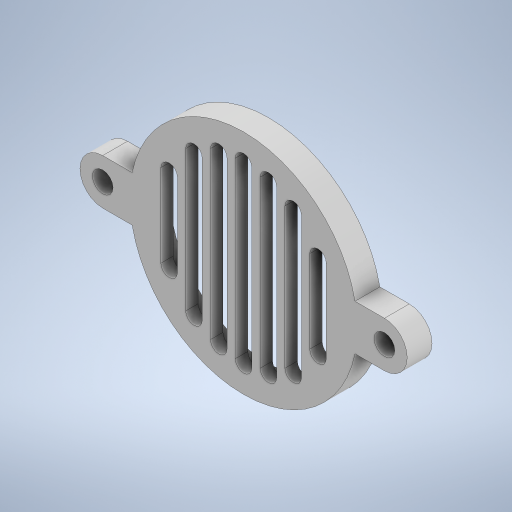
# Autodesk Inventor part: 스피커 홀더
Saved by Autodesk Inventor 2023 (Build 270158000, 158)
## iProperties
Created: 2022-11-10
Part Number: 스피커 홀더
Material: 일반
Document SubType Name: Modeling
Designer: user
Density: 1 g/cm^3
Appearance: 기본값
Author: user
Autodesk Inventor part; units mm, degrees
ref_plane "YZ Plane" through (0, 0, 0) normal (1, 0, 0) x (0, 1, 0)
ref_plane "XZ Plane" through (0, 0, 0) normal (0, 1, 0) x (-1, 0, 0)
ref_plane "XY Plane" through (0, 0, 0) normal (0, 0, 1) x (1, 0, 0)
sketch "스케치1" plane through (0, 0, 0) normal (0, 0, 1) x (1, 0, 0)
  circle A0 centre (0, 0) radius 13.75
  circle A1 centre (17.0329, 0) radius 1.25
  circle A2 centre (17.0329, 0) radius 2.75
  line L0 (17.0329, 2.75) -> (13.4722, 2.75)
  line L1 (17.0329, -2.75) -> (13.4722, -2.75)
  line L2 (0, 0) -> (0, 3.2191)
  circle A3 centre (-17.0329, 0) radius 1.25
  circle A4 centre (-17.0329, 0) radius 2.75
  line L3 (-17.0329, 2.75) -> (-13.4722, 2.75)
  line L4 (-17.0329, -2.75) -> (-13.4722, -2.75)
  dimension "d0" = 27.5
  dimension "d1" = 2.5
  dimension "d2" = 5.5
  constraints: 10 end point, 6 point on circle, 6 symmetric about line, 5 centre point, 3 coincident, 1 horizontal, 1 vertical, 2 other
  measures "d0" diameter of A0
  measures "d1" diameter of A1
  measures "d2" diameter of A2
extrude "돌출1" add sketch "스케치1" along normal blind 3
sketch "스케치2" plane through (0, 0, 0) normal (0, 0, -1) x (-1, 0, 0)
  circle A0 centre (0, 0) radius 12
  dimension "d5" = 24
  constraints: 1 centre point, 1 coincident
  measures "d5" diameter of A0
extrude "돌출2" cut sketch "스케치2" against normal blind 1.5
sketch "스케치3" plane through (0, 0, 1.5) normal (0, 0, -1) x (-1, 0, 0)
  line L0 (0, 10.5) -> (0, -10.5) construction
  line L1 (-1, 10.5) -> (-1, -10.5)
  line L2 (1, -10.5) -> (1, 10.5)
  arc A0 (1, 10.5) -> (-1, 10.5) centre (0, 10.5) ccw
  arc A1 (-1, -10.5) -> (1, -10.5) centre (0, -10.5) ccw
  line L3 (3, -10) -> (3, 10) construction
  line L4 (4, -10) -> (4, 10)
  line L5 (2, 10) -> (2, -10)
  arc A2 (2, -10) -> (4, -10) centre (3, -10) ccw
  arc A3 (4, 10) -> (2, 10) centre (3, 10) ccw
  line L6 (6, -8.5) -> (6, 8.5) construction
  line L7 (7, -8.5) -> (7, 8.5)
  line L8 (5, 8.5) -> (5, -8.5)
  arc A4 (5, -8.5) -> (7, -8.5) centre (6, -8.5) ccw
  arc A5 (7, 8.5) -> (5, 8.5) centre (6, 8.5) ccw
  line L9 (9, -5) -> (9, 5) construction
  line L10 (10, -5) -> (10, 5)
  line L11 (8, 5) -> (8, -5)
  arc A6 (8, -5) -> (10, -5) centre (9, -5) ccw
  arc A7 (10, 5) -> (8, 5) centre (9, 5) ccw
  line L12 (-3, -10) -> (-3, 10) construction
  line L13 (-4, -10) -> (-4, 10)
  line L14 (-2, 10) -> (-2, -10)
  arc A8 (-4, -10) -> (-2, -10) centre (-3, -10) ccw
  arc A9 (-2, 10) -> (-4, 10) centre (-3, 10) ccw
  line L15 (-6, -8.5) -> (-6, 8.5) construction
  line L16 (-7, -8.5) -> (-7, 8.5)
  line L17 (-5, 8.5) -> (-5, -8.5)
  arc A10 (-7, -8.5) -> (-5, -8.5) centre (-6, -8.5) ccw
  arc A11 (-5, 8.5) -> (-7, 8.5) centre (-6, 8.5) ccw
  line L18 (-9, -5) -> (-9, 5) construction
  line L19 (-10, -5) -> (-10, 5)
  line L20 (-8, 5) -> (-8, -5)
  arc A12 (-10, -5) -> (-8, -5) centre (-9, -5) ccw
  arc A13 (-8, 5) -> (-10, 5) centre (-9, 5) ccw
  point P0 (0, 0)
  point P1 (3, 0)
  point P2 (6, 0)
  point P3 (9, 0)
  point P4 (-3, 0)
  point P5 (-6, 0)
  point P6 (-9, 0)
  dimension "d8" = 21
  dimension "d9" = 1
  dimension "d10" = 1
  dimension "d11" = 1
  dimension "d12" = 20
  dimension "d13" = 17
  dimension "d14" = 1
  dimension "d15" = 1
  dimension "d17" = 1
  dimension "d18" = 10
  dimension "d19" = 1
  constraints: 56 end point, 28 point on circle, 21 symmetric about line, 16 tangent, 14 centre point, 6 parallel, 4 midpoint, 3 horizontal alignment, 2 vertical, 6 other
  measures "d8" distance of L0.start L0.end
  measures "d9" radius of A0
  measures "d10" radius of A3
  measures "d11" radius of A5
  measures "d12" distance of L3.start L3.end
  measures "d13" distance of L6.start L6.end
  measures "d14" distance between parallel lines of L2 L5
  measures "d15" distance between parallel lines of L4 L8
  measures "d17" radius of A7
  measures "d18" distance of L9.start L9.end
  measures "d19" distance between parallel lines of L7 L11
extrude "돌출3" cut sketch "스케치3" against normal blind 1.5
